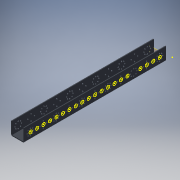
# Autodesk Inventor part: cut c channel
Saved by Autodesk Inventor 2016 (Build 200138000, 138)
## iProperties
Created: 2015-08-29
Part Number: cut c channel
Material: Generic
Description: CHANNEL - 416 MM
Document SubType Name: Modeling
Designer: PTC
Density: 1 g/cm^3
Appearance: Default
Sending System: Creo  TM  2.0  (c) 2012
PROJECT: FTC
PATTERN_NO: 6.0
PTC_MATERIAL_NAME: METAL_ALUMINIUM_5052
NIKCONFIGCOUNT: 1
KIT: TETRIX
Author: phi
Autodesk Inventor part; units mm, degrees
ref_plane "FRONT" through (0, 0, 0) normal (0, 0, 1) x (1, 0, 0)
ref_plane "TOP" through (0, 0, 0) normal (0, 1, 0) x (-1, 0, 0)
ref_plane "RIGHT" through (0, 0, 0) normal (1, 0, 0) x (0, 1, 0)
ref_plane "DTM1" through (0, 0, 16) normal (0, 0, 1) x (1, 0, 0)
ref_plane "Work Plane5" through (-14, 2, 16) normal (0, 0, 1) x (1, 0, 0)
sketch "Sketch2" plane through (-14, 2, 16) normal (0, 0, 1) x (1, 0, 0)
  arc A0 (-2, 0.5) -> (0.5, -2) centre (0.5, 0.5) ccw projected
  line L0 (-2, 0.5) -> (-2, 27.5) projected
  line L1 (0, 27.5) -> (0, 0) projected
  line L2 (-2, 30) -> (-2, 27.5) projected
  line L3 (0, 27.5) -> (0, 30) projected
  line L4 (0, 30) -> (-2, 30) projected
  line L5 (0, 0) -> (28, 0) projected
  line L6 (27.5, -2) -> (0.5, -2) projected
  arc A1 (27.5, -2) -> (30, 0.5) centre (27.5, 0.5) ccw projected
  line L7 (30, 27.5) -> (30, 0.5) projected
  line L8 (28, 0) -> (28, 27.5) projected
  line L9 (28, 30) -> (28, 27.5) projected
  line L10 (30, 30) -> (28, 30) projected
  line L11 (30, 27.5) -> (30, 30) projected
  point P0 (14, -2)
extrude "Extrusion1" add sketch "Sketch2" along normal blind 352
sketch "Sketch3" plane through (16, 2.5, 16) normal (1, 0, 0) x (0, 0, -1)
  circle A0 centre (-336, 21.5) radius 1.85 projected
  circle A1 centre (-341.6569, 19.1569) radius 1.85 projected
  circle A2 centre (-336, 13.5) radius 4 projected
  circle A3 centre (-344, 13.5) radius 1.85 projected
  circle A4 centre (-341.6569, 7.8431) radius 1.85 projected
  circle A5 centre (-336, 5.5) radius 1.85 projected
  circle A6 centre (-330.3431, 7.8431) radius 1.85 projected
  circle A7 centre (-328, 13.5) radius 1.85 projected
  circle A8 centre (-330.3431, 19.1569) radius 1.85 projected
  circle A9 centre (-320, 13.5) radius 4 projected
  circle A10 centre (-312, 13.5) radius 1.85 projected
  circle A11 centre (-304, 21.5) radius 1.85 projected
  circle A12 centre (-304, 13.5) radius 4 projected
  circle A13 centre (-304, 5.5) radius 1.85 projected
  circle A14 centre (-296, 13.5) radius 1.85 projected
  circle A15 centre (-288, 13.5) radius 4 projected
  circle A16 centre (-272, 13.5) radius 4 projected
  circle A17 centre (-266.3431, 19.1569) radius 1.85 projected
  circle A18 centre (-272, 21.5) radius 1.85 projected
  circle A19 centre (-277.6569, 19.1569) radius 1.85 projected
  circle A20 centre (-280, 13.5) radius 1.85 projected
  circle A21 centre (-277.6569, 7.8431) radius 1.85 projected
  circle A22 centre (-272, 5.5) radius 1.85 projected
  circle A23 centre (-266.3431, 7.8431) radius 1.85 projected
  circle A24 centre (-264, 13.5) radius 1.85 projected
  circle A25 centre (-256, 13.5) radius 4 projected
  circle A26 centre (-248, 13.5) radius 1.85 projected
  circle A27 centre (-240, 13.5) radius 4 projected
  circle A28 centre (-240, 21.5) radius 1.85 projected
  circle A29 centre (-232, 13.5) radius 1.85 projected
  circle A30 centre (-240, 5.5) radius 1.85 projected
  circle A31 centre (-213.6569, 7.8431) radius 1.85 projected
  circle A32 centre (-216, 13.5) radius 1.85 projected
  circle A33 centre (-213.6569, 19.1569) radius 1.85 projected
  circle A34 centre (-208, 21.5) radius 1.85 projected
  circle A35 centre (-202.3431, 19.1569) radius 1.85 projected
  circle A36 centre (-200, 13.5) radius 1.85 projected
  circle A37 centre (-202.3431, 7.8431) radius 1.85 projected
  circle A38 centre (-208, 5.5) radius 1.85 projected
  circle A39 centre (-224, 13.5) radius 4 projected
  circle A40 centre (-208, 13.5) radius 4 projected
  circle A41 centre (-192, 13.5) radius 4 projected
  circle A42 centre (-184, 13.5) radius 1.85 projected
  circle A43 centre (-176, 13.5) radius 4 projected
  circle A44 centre (-176, 21.5) radius 1.85 projected
  circle A45 centre (-168, 13.5) radius 1.85 projected
  circle A46 centre (-176, 5.5) radius 1.85 projected
  circle A47 centre (-160, 13.5) radius 4 projected
  circle A48 centre (-152, 13.5) radius 1.85 projected
  circle A49 centre (-144, 13.5) radius 4 projected
  circle A50 centre (-144, 21.5) radius 1.85 projected
  circle A51 centre (-149.6569, 19.1569) radius 1.85 projected
  circle A52 centre (-149.6569, 7.8431) radius 1.85 projected
  circle A53 centre (-144, 5.5) radius 1.85 projected
  circle A54 centre (-138.3431, 7.8431) radius 1.85 projected
  circle A55 centre (-136, 13.5) radius 1.85 projected
  circle A56 centre (-138.3431, 19.1569) radius 1.85 projected
  circle A57 centre (-128, 13.5) radius 4 projected
  circle A58 centre (-120, 13.5) radius 1.85 projected
  circle A59 centre (-112, 13.5) radius 4 projected
  circle A60 centre (-112, 21.5) radius 1.85 projected
  circle A61 centre (-104, 13.5) radius 1.85 projected
  circle A62 centre (-112, 5.5) radius 1.85 projected
  circle A63 centre (-96, 13.5) radius 4 projected
  circle A64 centre (-88, 13.5) radius 1.85 projected
  circle A65 centre (-85.6569, 19.1569) radius 1.85 projected
  circle A66 centre (-80, 21.5) radius 1.85 projected
  circle A67 centre (-74.3431, 19.1569) radius 1.85 projected
  circle A68 centre (-72, 13.5) radius 1.85 projected
  circle A69 centre (-74.3431, 7.8431) radius 1.85 projected
  circle A70 centre (-80, 5.5) radius 1.85 projected
  circle A71 centre (-85.6569, 7.8431) radius 1.85 projected
  circle A72 centre (-80, 13.5) radius 4 projected
  circle A73 centre (-64, 13.5) radius 4 projected
  circle A74 centre (-56, 13.5) radius 1.85 projected
  circle A75 centre (-48, 13.5) radius 4 projected
  circle A76 centre (-48, 21.5) radius 1.85 projected
  circle A77 centre (-40, 13.5) radius 1.85 projected
  circle A78 centre (-48, 5.5) radius 1.85 projected
  circle A79 centre (-32, 13.5) radius 4 projected
  circle A80 centre (-24, 13.5) radius 1.85 projected
  circle A81 centre (-21.6569, 19.1569) radius 1.85 projected
  circle A82 centre (-16, 21.5) radius 1.85 projected
  circle A83 centre (-10.3431, 19.1569) radius 1.85 projected
  circle A84 centre (-8, 13.5) radius 1.85 projected
  circle A85 centre (-10.3431, 7.8431) radius 1.85 projected
  circle A86 centre (-16, 5.5) radius 1.85 projected
  circle A87 centre (-21.6569, 7.8431) radius 1.85 projected
  circle A88 centre (-16, 13.5) radius 4 projected
  point P0 (16, -2.5)
hole "Hole1" at (16, 16, 360) at (16, 21.6569, 357.6569) at (16, 24, 352) at (16, 21.6569, 346.3431) at (16, 16, 344) at (16, 10.3431, 346.3431) at (16, 8, 352) at (16, 10.3431, 357.6569) at (16, 16, 328) at (16, 24, 320) at (16, 16, 312) at (16, 8, 320) at (16, 16, 296) at (16, 21.6569, 293.6569) at (16, 24, 288) at (16, 16, 280) at (16, 21.6569, 282.3431) at (16, 10.3431, 282.3431) at (16, 8, 288) at (16, 10.3431, 293.6569) at (16, 16, 264) at (16, 24, 256) at (16, 16, 248) at (16, 8, 256) at (16, 16, 232) at (16, 21.6569, 229.6569) at (16, 24, 224) at (16, 21.6569, 218.3431) at (16, 16, 216) at (16, 10.3431, 218.3431) at (16, 8, 224) at (16, 10.3431, 229.6569) at (16, 16, 200) at (16, 24, 192) at (16, 16, 184) at (16, 8, 192) at (16, 16, 168) at (16, 21.6569, 165.6569) at (16, 24, 160) at (16, 21.6569, 154.3431) at (16, 16, 152) at (16, 10.3431, 154.3431) at (16, 8, 160) at (16, 10.3431, 165.6569) at (16, 16, 136) at (16, 24, 128) at (16, 16, 120) at (16, 8, 128) at (16, 16, 104) at (16, 21.6569, 101.6569) direction (-1, 0, 0) diameter 3.7 end through all and at (16, 24, 96) (16, 21.6569, 90.3431) (16, 16, 88) (16, 10.3431, 90.3431) (16, 8, 96) (16, 10.3431, 101.6569) (16, 16, 72) (16, 24, 64) (16, 16, 56) (16, 8, 64) (16, 24, 32) (16, 21.6569, 37.6569) (16, 16, 40) (16, 10.3431, 37.6569) (16, 8, 32) (16, 10.3431, 26.3431) (16, 16, 24) (16, 21.6569, 26.3431)
sketch "Sketch4" plane through (16, 2.5, 16) normal (1, 0, 0) x (0, 0, -1)
  circle A0 centre (-336, 13.5) radius 4 projected
  circle A1 centre (-320, 13.5) radius 4 projected
  circle A2 centre (-304, 13.5) radius 4 projected
  circle A3 centre (-288, 13.5) radius 4 projected
  circle A4 centre (-272, 13.5) radius 4 projected
  circle A5 centre (-256, 13.5) radius 4 projected
  circle A6 centre (-240, 13.5) radius 4 projected
  circle A7 centre (-224, 13.5) radius 4 projected
  circle A8 centre (-208, 13.5) radius 4 projected
  circle A9 centre (-192, 13.5) radius 4 projected
  circle A10 centre (-176, 13.5) radius 4 projected
  circle A11 centre (-160, 13.5) radius 4 projected
  circle A12 centre (-144, 13.5) radius 4 projected
  circle A13 centre (-128, 13.5) radius 4 projected
  circle A14 centre (-112, 13.5) radius 4 projected
  circle A15 centre (-96, 13.5) radius 4 projected
  circle A16 centre (-64, 13.5) radius 4 projected
  circle A17 centre (-48, 13.5) radius 4 projected
  circle A18 centre (-32, 13.5) radius 4 projected
  circle A19 centre (-16, 13.5) radius 4 projected
  circle A20 centre (-80, 13.5) radius 4 projected
  point P0 (16, -2.5)
hole "Hole2" at (16, 16, 352) at (16, 16, 336) at (16, 16, 320) at (16, 16, 304) at (16, 16, 288) at (16, 16, 272) at (16, 16, 256) at (16, 16, 240) at (16, 16, 224) at (16, 16, 192) at (16, 16, 208) at (16, 16, 176) at (16, 16, 160) at (16, 16, 144) at (16, 16, 128) at (16, 16, 112) at (16, 16, 80) at (16, 16, 64) at (16, 16, 48) at (16, 16, 32) at (16, 16, 96) direction (-1, 0, 0) diameter 8 end through all
sketch "Sketch5" plane through (-13.5, 0, 16) normal (0, -1, 0) x (1, 0, 0)
  line L0 (-0.5, -64) -> (27.5, -64) projected
  line L1 (27.5, 352) -> (27.5, -64) projected
  line L2 (-0.5, 352) -> (27.5, 352) projected
  line L3 (-0.5, 352) -> (-0.5, -64) projected
  circle A0 centre (13.5, -48) radius 4 projected
  circle A1 centre (5.5, -48) radius 1.85 projected
  circle A2 centre (7.8431, -42.3431) radius 1.85 projected
  circle A3 centre (13.5, -40) radius 1.85 projected
  circle A4 centre (19.1569, -42.3431) radius 1.85 projected
  circle A5 centre (21.5, -48) radius 1.85 projected
  circle A6 centre (19.1569, -53.6569) radius 1.85 projected
  circle A7 centre (13.5, -56) radius 1.85 projected
  circle A8 centre (7.8431, -53.6569) radius 1.85 projected
  circle A9 centre (13.5, 16) radius 4 projected
  circle A10 centre (5.5, 16) radius 1.85 projected
  circle A11 centre (7.8431, 21.6569) radius 1.85 projected
  circle A12 centre (13.5, 24) radius 1.85 projected
  circle A13 centre (19.1569, 21.6569) radius 1.85 projected
  circle A14 centre (21.5, 16) radius 1.85 projected
  circle A15 centre (19.1569, 10.3431) radius 1.85 projected
  circle A16 centre (13.5, 8) radius 1.85 projected
  circle A17 centre (7.8431, 10.3431) radius 1.85 projected
  circle A18 centre (13.5, 80) radius 4 projected
  circle A19 centre (5.5, 80) radius 1.85 projected
  circle A20 centre (7.8431, 85.6569) radius 1.85 projected
  circle A21 centre (13.5, 88) radius 1.85 projected
  circle A22 centre (19.1569, 85.6569) radius 1.85 projected
  circle A23 centre (21.5, 80) radius 1.85 projected
  circle A24 centre (19.1569, 74.3431) radius 1.85 projected
  circle A25 centre (13.5, 72) radius 1.85 projected
  circle A26 centre (7.8431, 74.3431) radius 1.85 projected
  circle A27 centre (13.5, 144) radius 4 projected
  circle A28 centre (5.5, 144) radius 1.85 projected
  circle A29 centre (7.8431, 149.6569) radius 1.85 projected
  circle A30 centre (13.5, 152) radius 1.85 projected
  circle A31 centre (19.1569, 149.6569) radius 1.85 projected
  circle A32 centre (21.5, 144) radius 1.85 projected
  circle A33 centre (19.1569, 138.3431) radius 1.85 projected
  circle A34 centre (13.5, 136) radius 1.85 projected
  circle A35 centre (7.8431, 138.3431) radius 1.85 projected
  circle A36 centre (13.5, 208) radius 4 projected
  circle A37 centre (5.5, 208) radius 1.85 projected
  circle A38 centre (7.8431, 213.6569) radius 1.85 projected
  circle A39 centre (13.5, 216) radius 1.85 projected
  circle A40 centre (19.1569, 213.6569) radius 1.85 projected
  circle A41 centre (21.5, 208) radius 1.85 projected
  circle A42 centre (19.1569, 202.3431) radius 1.85 projected
  circle A43 centre (13.5, 200) radius 1.85 projected
  circle A44 centre (7.8431, 202.3431) radius 1.85 projected
  circle A45 centre (13.5, 272) radius 4 projected
  circle A46 centre (5.5, 272) radius 1.85 projected
  circle A47 centre (7.8431, 277.6569) radius 1.85 projected
  circle A48 centre (13.5, 280) radius 1.85 projected
  circle A49 centre (19.1569, 277.6569) radius 1.85 projected
  circle A50 centre (21.5, 272) radius 1.85 projected
  circle A51 centre (19.1569, 266.3431) radius 1.85 projected
  circle A52 centre (13.5, 264) radius 1.85 projected
  circle A53 centre (7.8431, 266.3431) radius 1.85 projected
  circle A54 centre (13.5, 336) radius 4 projected
  circle A55 centre (5.5, 336) radius 1.85 projected
  circle A56 centre (7.8431, 341.6569) radius 1.85 projected
  circle A57 centre (13.5, 344) radius 1.85 projected
  circle A58 centre (19.1569, 341.6569) radius 1.85 projected
  circle A59 centre (21.5, 336) radius 1.85 projected
  circle A60 centre (19.1569, 330.3431) radius 1.85 projected
  circle A61 centre (13.5, 328) radius 1.85 projected
  circle A62 centre (7.8431, 330.3431) radius 1.85 projected
  circle A63 centre (13.5, -16) radius 4 projected
  circle A64 centre (5.5, -16) radius 1.85 projected
  circle A65 centre (13.5, -8) radius 1.85 projected
  circle A66 centre (21.5, -16) radius 1.85 projected
  circle A67 centre (13.5, -24) radius 1.85 projected
  circle A68 centre (13.5, 48) radius 4 projected
  circle A69 centre (5.5, 48) radius 1.85 projected
  circle A70 centre (13.5, 56) radius 1.85 projected
  circle A71 centre (21.5, 48) radius 1.85 projected
  circle A72 centre (13.5, 40) radius 1.85 projected
  circle A73 centre (13.5, 112) radius 4 projected
  circle A74 centre (5.5, 112) radius 1.85 projected
  circle A75 centre (13.5, 120) radius 1.85 projected
  circle A76 centre (21.5, 112) radius 1.85 projected
  circle A77 centre (13.5, 104) radius 1.85 projected
  circle A78 centre (13.5, 176) radius 4 projected
  circle A79 centre (5.5, 176) radius 1.85 projected
  circle A80 centre (13.5, 184) radius 1.85 projected
  circle A81 centre (21.5, 176) radius 1.85 projected
  circle A82 centre (13.5, 168) radius 1.85 projected
  circle A83 centre (13.5, 240) radius 4 projected
  circle A84 centre (5.5, 240) radius 1.85 projected
  circle A85 centre (13.5, 248) radius 1.85 projected
  circle A86 centre (21.5, 240) radius 1.85 projected
  circle A87 centre (13.5, 232) radius 1.85 projected
  circle A88 centre (13.5, 304) radius 4 projected
  circle A89 centre (5.5, 304) radius 1.85 projected
  circle A90 centre (13.5, 312) radius 1.85 projected
  circle A91 centre (21.5, 304) radius 1.85 projected
  circle A92 centre (13.5, 296) radius 1.85 projected
  circle A93 centre (13.5, -32) radius 4 projected
  circle A94 centre (13.5, 0) radius 4 projected
  circle A95 centre (13.5, 32) radius 4 projected
  circle A96 centre (13.5, 64) radius 4 projected
  circle A97 centre (13.5, 96) radius 4 projected
  circle A98 centre (13.5, 128) radius 4 projected
  circle A99 centre (13.5, 160) radius 4 projected
  circle A100 centre (13.5, 192) radius 4 projected
  circle A101 centre (13.5, 224) radius 4 projected
  circle A102 centre (13.5, 256) radius 4 projected
  circle A103 centre (13.5, 288) radius 4 projected
  circle A104 centre (13.5, 320) radius 4 projected
  point P0 (13.5, -16)
hole "Hole3" at (8, 0, 32) at (5.6569, 0, 26.3431) at (0, 0, 24) at (-5.6569, 0, 26.3431) at (-8, 0, 32) at (-5.6569, 0, 37.6569) at (5.6569, 0, 37.6569) at (0, 0, 40) at (0, 0, 56) at (8, 0, 64) at (0, 0, 72) at (-8, 0, 64) at (0, 0, 88) at (5.6569, 0, 90.3431) at (8, 0, 96) at (5.6569, 0, 101.6569) at (0, 0, 104) at (-5.6569, 0, 101.6569) at (-8, 0, 96) at (-5.6569, 0, 90.3431) at (0, 0, 120) at (8, 0, 128) at (0, 0, 136) at (-8, 0, 128) at (0, 0, 152) at (5.6569, 0, 154.3431) at (8, 0, 160) at (5.6569, 0, 165.6569) at (0, 0, 168) at (-5.6569, 0, 165.6569) at (-8, 0, 160) at (-5.6569, 0, 154.3431) at (0, 0, 184) at (8, 0, 192) at (0, 0, 200) at (-8, 0, 192) at (0, 0, 216) at (5.6569, 0, 218.3431) at (8, 0, 224) at (5.6569, 0, 229.6569) at (0, 0, 232) at (-5.6569, 0, 229.6569) at (-8, 0, 224) at (-5.6569, 0, 218.3431) at (0, 0, 248) at (8, 0, 256) at (0, 0, 264) at (-8, 0, 256) at (0, 0, 280) at (5.6569, 0, 282.3431) direction (0, 1, 0) diameter 3.7 end through all and at (8, 0, 288) (5.6569, 0, 293.6569) (0, 0, 296) (-5.6569, 0, 293.6569) (-8, 0, 288) (-5.6569, 0, 282.3431) (0, 0, 312) (0, 0, 328) (-8, 0, 320) (8, 0, 320) (0, 0, 344) (5.6569, 0, 346.3431) (8, 0, 352) (5.6569, 0, 357.6569) (0, 0, 360) (-5.6569, 0, 357.6569) (-8, 0, 352) (-5.6569, 0, 346.3431)
sketch "Sketch6" plane through (-13.5, 0, 16) normal (0, -1, 0) x (1, 0, 0)
  circle A0 centre (13.5, 336) radius 4 projected
  circle A1 centre (13.5, 320) radius 4 projected
  circle A2 centre (13.5, 304) radius 4 projected
  circle A3 centre (13.5, 288) radius 4 projected
  circle A4 centre (13.5, 272) radius 4 projected
  circle A5 centre (13.5, 256) radius 4 projected
  circle A6 centre (13.5, 240) radius 4 projected
  circle A7 centre (13.5, 224) radius 4 projected
  circle A8 centre (13.5, 208) radius 4 projected
  circle A9 centre (13.5, 192) radius 4 projected
  circle A10 centre (13.5, 176) radius 4 projected
  circle A11 centre (13.5, 160) radius 4 projected
  circle A12 centre (13.5, 144) radius 4 projected
  circle A13 centre (13.5, 128) radius 4 projected
  circle A14 centre (13.5, 112) radius 4 projected
  circle A15 centre (13.5, 96) radius 4 projected
  circle A16 centre (13.5, 80) radius 4 projected
  circle A17 centre (13.5, 64) radius 4 projected
  circle A18 centre (13.5, 48) radius 4 projected
  circle A19 centre (13.5, 32) radius 4 projected
  circle A20 centre (13.5, 16) radius 4 projected
  point P0 (13.5, -16)
hole "Hole4" at (0, 0, 352) at (0, 0, 336) at (0, 0, 320) at (0, 0, 304) at (0, 0, 288) at (0, 0, 272) at (0, 0, 256) at (0, 0, 240) at (0, 0, 224) at (0, 0, 208) at (0, 0, 192) at (0, 0, 176) at (0, 0, 160) at (0, 0, 144) at (0, 0, 128) at (0, 0, 112) at (0, 0, 96) at (0, 0, 80) at (0, 0, 64) at (0, 0, 48) at (0, 0, 32) direction (0, 1, 0) diameter 8 end through all
body "Solid2"
